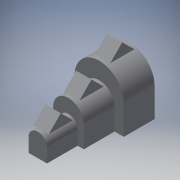
# Autodesk Inventor part: Tail6
Saved by Autodesk Inventor 2016 (Build 200138000, 138)
## iProperties
Created: 2017-03-09
Part Number: Tail6
Material: Generic
Document SubType Name: Modeling
Designer: Owner
Density: 1 g/cm^3
Appearance: Default
Author: Owner
Autodesk Inventor part; units mm, degrees
ref_plane "YZ Plane" through (0, 0, 0) normal (1, 0, 0) x (0, 1, 0)
ref_plane "XZ Plane" through (0, 0, 0) normal (0, 1, 0) x (-1, 0, 0)
ref_plane "XY Plane" through (0, 0, 0) normal (0, 0, 1) x (1, 0, 0)
sketch "Sketch1" plane through (0, 0, 0) normal (0, 0, 1) x (1, 0, 0)
  line L0 (6.35, -38.0962) -> (6.35, -43.1) projected
  line L1 (6.35, -43.1) -> (24.13, -43.1) projected
  line L2 (24.13, -43.1) -> (24.13, 0) projected
  arc A0 (24.13, 0) -> (-24.13, 0) centre (0, 0) ccw projected
  line L3 (-24.13, 0) -> (-24.13, -43.1) projected
  line L4 (-24.13, -43.1) -> (-6.35, -43.1) projected
  line L5 (-6.35, -43.1) -> (-6.35, -38.0962) projected
  line L6 (-6.35, -38.0962) -> (6.35, -38.0962) projected
  line L7 (20.32, -43.1) -> (-20.32, -43.1)
  line L8 (0, 0) -> (0, -19.05)
  circle A1 centre (0, -19.05) radius 20.32
  line L9 (-20.32, -19.05) -> (20.32, -19.05)
  line L10 (20.32, -19.05) -> (20.32, -43.1)
  line L11 (20.32, -43.1) -> (-20.32, -43.1)
  line L12 (-20.32, -43.1) -> (-20.32, -19.05)
  dimension "d26" = 40.64
  dimension "d25" = 19.05
  constraints: 12 end point, 2 coincident, 2 parallel, 1 horizontal, 1 horizontal alignment, 1 perpendicular, 1 point on line, 1 vertical, 2 other
  measures "d25" distance of L8.start L8.end
extrude "Extrusion1" add sketch "Sketch1" along normal blind 25.4 contours L6 L5 A1 L9 L0 | L0 A1 L5 L6 | A1 L10 L1 L0 | L0 L7 L5 A1 | L5 L4 L12 A1 | L9 A1
sketch "Sketch2" plane through (0, 0, 0) normal (0, 0, -1) x (-1, 0, 0)
  line L0 (6.35, -43.1) -> (-6.35, -43.1) projected
  line L1 (-6.35, -43.1) -> (-6.35, -38.0962) projected
  line L2 (-6.35, -38.0962) -> (6.35, -38.0962) projected
  line L3 (6.35, -38.0962) -> (6.35, -43.1) projected
  line L4 (-6.35, -38.0962) -> (6.35, -38.0962)
  line L5 (6.35, -38.0962) -> (6.35, -33.0924)
  line L6 (6.35, -33.0924) -> (-6.35, -33.0924)
  line L7 (-6.35, -33.0924) -> (-6.35, -38.0962)
  point P0 (0, 0)
  dimension "d3" = 5.0038
  constraints: 8 end point, 2 parallel, 1 horizontal, 1 perpendicular
  measures "d3" distance of L4.end L5.end
extrude "Extrusion2" add sketch "Sketch2" along normal blind 10.16 contours L2 L7 L6 L5
sketch "Sketch3" plane through (-6.35, -33.0924, 0) normal (0, 1, 0) x (1, 0, 0)
  line L0 (6.35, 10.2144) -> (6.35, 6.4044)
  circle A0 centre (6.35, 6.4044) radius 2.25
  point P0 (6.35, 0)
  dimension "d6" = 3.81
  dimension "d7" = 4.5
  constraints: 2 end point, 1 centre point, 1 coincident, 1 vertical
  measures "d6" distance of L0.start L0.end
  measures "d7" diameter of A0
extrude "Extrusion3" cut sketch "Sketch3" against normal blind 10.16
sketch "Sketch4" plane through (0, 0, 25.4) normal (0, 0, 1) x (1, 0, 0)
  arc A0 (20.32, -19.05) -> (-20.32, -19.05) centre (0, -19.05) ccw projected
  line L0 (0, -19.05) -> (0, -25.4)
  circle A1 centre (0, -25.4) radius 12.7
  line L1 (-12.7, -25.4) -> (12.7, -25.4)
  line L2 (12.7, -25.4) -> (12.7, -42.8987)
  line L3 (12.7, -42.8987) -> (-12.7, -42.8987)
  line L4 (-12.7, -42.8987) -> (-12.7, -25.4)
  point P0 (0, 0)
  dimension "d28" = 25.4
  dimension "d27" = 6.35
  constraints: 10 end point, 2 parallel, 1 coincident, 1 horizontal, 1 horizontal alignment, 1 perpendicular, 1 vertical, 2 other
  measures "d27" distance of L0.start L0.end
extrude "Extrusion4" add sketch "Sketch4" along normal blind 25.4
sketch "Sketch5" plane through (0, 0, 50.8) normal (0, 0, 1) x (1, 0, 0)
  arc A0 (12.7, -25.4) -> (-12.7, -25.4) centre (0, -25.4) ccw projected
  line L0 (0, -25.4) -> (0, -31.75)
  circle A1 centre (0, -31.75) radius 7.62
  line L1 (-20.32, -43.1) -> (20.32, -43.1) projected
  line L2 (-7.62, -31.75) -> (7.62, -31.75)
  line L3 (7.62, -31.75) -> (7.62, -43.1)
  line L4 (7.62, -43.1) -> (-7.62, -43.1)
  line L5 (-7.62, -43.1) -> (-7.62, -31.75)
  point P0 (0, 0)
  dimension "d30" = 15.24
  dimension "d29" = 6.35
  constraints: 10 end point, 2 parallel, 1 coincident, 1 horizontal, 1 horizontal alignment, 1 perpendicular, 1 point on line, 1 vertical, 2 other
  measures "d29" distance of L0.start L0.end
extrude "Extrusion5" add sketch "Sketch5" along normal blind 25.4
ref_plane "Work Plane1" through (0, -43.1, 0) normal (-1, 0, 0) x (0, 0, 1)
sketch "Sketch8" plane through (0, -43.1, 0) normal (-1, 0, 0) x (0, 0, 1)
  line L0 (0, 44.37) -> (0, 24.05) projected
  line L1 (0, 44.37) -> (2.7051, 44.37)
  line L2 (0, 44.37) -> (25.4, 44.37) projected
  line L3 (2.7051, 44.37) -> (22.6949, 44.37)
  line L4 (22.6949, 44.37) -> (12.6873, 44.37)
  line L5 (12.6873, 44.37) -> (12.6873, 54.3776)
  line L6 (12.6873, 54.3776) -> (22.6949, 44.37)
  line L7 (12.6873, 54.3776) -> (2.6797, 44.37)
  line L8 (12.6873, 54.3776) -> (2.6797, 44.37)
  line L9 (2.6797, 44.37) -> (22.6949, 44.37)
  point P0 (0, 43.1)
  dimension "d32" = 2.7051
  dimension "d33" = 19.9898
  dimension "d34" = 10.0076
  dimension "d35" = 10.0076
  constraints: 16 end point, 4 point on line, 2 perpendicular, 1 horizontal
  measures "d32" distance of L0.start L1.end
  measures "d33" distance of L1.end L3.end
  measures "d34" distance of L3.end L4.end
  measures "d35" distance of L4.end L5.end
extrude "Extrusion8" add sketch "Sketch8" along normal mid plane 12.7
sketch "Sketch9" plane through (0, -43.1, 0) normal (-1, 0, 0) x (0, 0, 1)
  line L0 (25.4, 30.4) -> (50.8, 30.4) projected
  line L1 (25.4, 30.4) -> (28.1051, 30.4)
  line L2 (28.1051, 30.4) -> (48.0949, 30.4)
  line L3 (48.0949, 30.4) -> (38.0873, 30.4)
  line L4 (38.0873, 30.4) -> (38.0873, 40.4076)
  line L5 (38.0873, 40.4076) -> (48.0949, 30.4)
  line L6 (38.0873, 40.4076) -> (28.1051, 30.4)
  point P0 (0, 43.1)
  dimension "d38" = 2.7051
  dimension "d39" = 19.9898
  dimension "d40" = 10.0076
  dimension "d41" = 10.0076
  constraints: 12 end point, 4 point on line, 1 perpendicular
  measures "d38" distance of L1.start L1.end
  measures "d39" distance of L1.end L2.end
  measures "d40" distance of L2.end L3.end
  measures "d41" distance of L3.end L4.end
extrude "Extrusion9" add sketch "Sketch9" along normal mid plane 12.7
sketch "Sketch10" plane through (0, -43.1, 0) normal (-1, 0, 0) x (0, 0, 1)
  line L0 (50.8, 18.97) -> (76.2, 18.97) projected
  line L1 (50.8, 18.97) -> (53.5051, 18.97)
  line L2 (53.5051, 18.97) -> (73.4949, 18.97)
  line L3 (73.4949, 18.97) -> (63.4873, 18.97)
  line L4 (63.4873, 18.97) -> (63.4873, 28.9776)
  line L5 (63.4873, 28.9776) -> (73.4949, 18.97)
  line L6 (63.4873, 28.9776) -> (53.5051, 18.97)
  point P0 (0, 43.1)
  dimension "d44" = 2.7051
  dimension "d45" = 19.9898
  dimension "d46" = 10.0076
  dimension "d47" = 10.0076
  constraints: 12 end point, 4 point on line, 1 perpendicular
  measures "d44" distance of L1.start L1.end
  measures "d45" distance of L1.end L2.end
  measures "d46" distance of L2.end L3.end
  measures "d47" distance of L3.end L4.end
extrude "Extrusion10" add sketch "Sketch10" along normal mid plane 12.7
sketch "Sketch11" plane through (-12.7, -42.8987, 25.4) normal (0, -1, 0) x (1, 0, 0)
  line L0 (25.4, 0) -> (0, 0) projected
  line L1 (25.4, 0) -> (25.4, 25.4) projected
  line L2 (20.32, 25.4) -> (25.4, 25.4) projected
  line L3 (5.08, 25.4) -> (20.32, 25.4) projected
  line L4 (0, 25.4) -> (5.08, 25.4) projected
  line L5 (0, 0) -> (0, 25.4) projected
  point P0 (12.7, -25.4)
extrude "Extrusion11" add sketch "Sketch11" along normal blind 0.2
sketch "Sketch12" plane through (0, 0, 0) normal (0, 0, -1) x (-1, 0, 0)
  ellipse E0 centre (-8.9523, -27.5683) end of major axis (-8.9523, -28.8129) minor radius 1.2444 projected
  ellipse E1 centre (7.1732, -27.5683) end of major axis (7.1732, -28.8129) minor radius 1.2444 projected
  line L0 (-8.9523, -27.5683) -> (-7.9523, -27.5683)
  line L1 (7.1732, -27.5683) -> (6.1732, -27.5683)
  circle A0 centre (-7.9523, -27.5683) radius 1.2446
  circle A1 centre (6.1732, -27.5683) radius 1.2446
  point P0 (0, 0)
  dimension "d52" = 1
  dimension "d53" = 1
  dimension "d54" = 2.4892
  dimension "d55" = 2.4892
  constraints: 4 end point, 2 centre point, 2 coincident, 2 horizontal, 2 other
  measures "d52" distance of L0.start L0.end
  measures "d53" distance of L1.start L1.end
  measures "d54" diameter of A0
  measures "d55" diameter of A1
extrude "Extrusion12" cut sketch "Sketch12" against normal blind 25.4 contours A0 E0 | E0 A0 | A1 E1 | E1 A1 picked at (-8.6972, -27.743) picked at (-7.0538, -27.6701) picked at (6.9181, -27.3936) picked at (5.2747, -27.4665)
body "Solid1"
